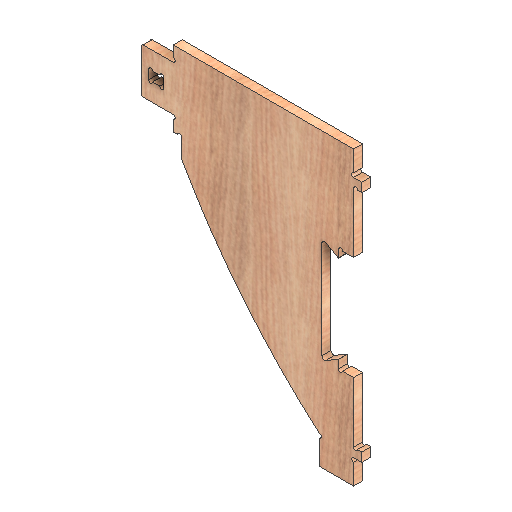
# Autodesk Inventor part: Support F
Saved by Autodesk Inventor 2021 (Build 250183000, 183)
## iProperties
Created: 2020-05-09
Part Number: Support F
Material: Wood (Birch)
Document SubType Name: Modeling
Designer: Dan Wikman
Density: 0.55 g/cm^3
Appearance: Birch - Natural Polished
Mass: 1365.58 g
Surface Area: 3158.08 cm^2
Volume: 2482.87 cm^3
Autodesk Inventor part; units mm, degrees
ref_plane "YZ Plane" through (0, 0, 0) normal (1, 0, 0) x (0, 1, 0)
ref_plane "XZ Plane" through (0, 0, 0) normal (0, 1, 0) x (-1, 0, 0)
ref_plane "XY Plane" through (0, 0, 0) normal (0, 0, 1) x (1, 0, 0)
sketch "CONTOURS" plane through (0, 0, 0) normal (0, 0, 1) x (1, 0, 0)
  arc A0 (2413.107, 689.155) -> (2421.107, 689.155) centre (2417.107, 689.155) ccw
  line L0 (2421.107, 689.155) -> (2429.607, 689.155)
  line L1 (2429.607, 689.155) -> (2429.607, 671.155)
  line L2 (2429.607, 671.155) -> (2413.107, 671.155)
  arc A1 (2413.107, 671.155) -> (2413.107, 663.155) centre (2413.107, 667.155) ccw
  line L3 (2413.107, 663.155) -> (2413.107, 622.1071)
  line L4 (2413.107, 622.1071) -> (2345.607, 622.1071)
  line L5 (2345.607, 622.1071) -> (2345.607, 670.507)
  arc A2 (2345.607, 670.507) -> (2345.607, 678.507) centre (2345.607, 674.507) ccw
  arc A3 (2070.607, 1014.7918) -> (2345.607, 678.507) centre (3181.8457, 1642.9335) ccw
  line L6 (2070.607, 1014.7918) -> (2070.607, 1053.1873)
  arc A4 (2070.607, 1053.1873) -> (2062.607, 1053.1873) centre (2066.607, 1053.1873) ccw
  line L7 (2062.607, 1053.1873) -> (2055.607, 1053.1873)
  line L8 (2055.607, 1053.1873) -> (2054.248, 1053.1873)
  line L9 (2054.248, 1053.1873) -> (2054.248, 1075.1087)
  arc A5 (2054.248, 1075.1087) -> (2054.248, 1083.1087) centre (2054.248, 1079.1087) ccw
  line L10 (2054.248, 1083.1087) -> (1994.248, 1083.1087)
  arc A6 (1990.248, 1087.1087) -> (1994.248, 1083.1087) centre (1994.248, 1087.1087) ccw
  line L11 (1990.248, 1087.1087) -> (1990.248, 1169.1087)
  arc A7 (1994.248, 1173.1087) -> (1990.248, 1169.1087) centre (1994.248, 1169.1087) ccw
  line L12 (1994.248, 1173.1087) -> (2054.248, 1173.1087)
  arc A8 (2054.248, 1173.1087) -> (2054.248, 1181.1087) centre (2054.248, 1177.1087) ccw
  line L13 (2054.248, 1181.1087) -> (2054.248, 1203.107)
  line L14 (2054.248, 1203.107) -> (2413.107, 1203.107)
  line L15 (2413.107, 1203.107) -> (2413.107, 1162.0591)
  arc A9 (2413.107, 1162.0591) -> (2413.107, 1154.0591) centre (2413.107, 1158.0591) ccw
  line L16 (2413.107, 1154.0591) -> (2429.607, 1154.0591)
  line L17 (2429.607, 1154.0591) -> (2429.607, 1136.0591)
  line L18 (2429.607, 1136.0591) -> (2421.107, 1136.0591)
  arc A10 (2421.107, 1136.0591) -> (2413.107, 1136.0591) centre (2417.107, 1136.0591) ccw
  line L19 (2413.107, 1136.0591) -> (2413.107, 1016.107)
  line L20 (2413.107, 1016.107) -> (2391.107, 1016.107)
  arc A11 (2391.107, 1016.107) -> (2383.107, 1016.107) centre (2387.107, 1016.107) ccw
  line L21 (2383.107, 1016.107) -> (2383.107, 999.7176)
  line L22 (2383.107, 999.7176) -> (2382.8653, 999.8478)
  line L23 (2382.8653, 999.8478) -> (2382.6262, 999.9827)
  line L24 (2382.6262, 999.9827) -> (2357.4659, 1014.509)
  arc A12 (2357.4659, 1014.509) -> (2349.9659, 1010.1788) centre (2354.9659, 1010.1788) ccw
  line L25 (2349.9659, 1010.1788) -> (2349.9659, 815.0352)
  arc A13 (2349.9659, 815.0352) -> (2357.4659, 810.7051) centre (2354.9659, 815.0352) ccw
  line L26 (2357.4659, 810.7051) -> (2382.6262, 825.2314)
  line L27 (2382.6262, 825.2314) -> (2382.8653, 825.3663)
  line L28 (2382.8653, 825.3663) -> (2383.107, 825.4965)
  line L29 (2383.107, 825.4965) -> (2383.107, 809.1071)
  arc A14 (2383.107, 809.1071) -> (2391.107, 809.107) centre (2387.107, 809.107) ccw
  line L30 (2391.107, 809.107) -> (2413.107, 809.107)
  line L31 (2413.107, 809.107) -> (2413.107, 689.155)
  constraints: 64 end point, 30 point on circle, 15 centre point
sketch "HOLES" plane through (0, 0, 0) normal (0, 0, 1) x (1, 0, 0)
  arc A0 (2013.248, 1137.6087) -> (2005.248, 1137.6087) centre (2009.248, 1137.6087) ccw
  line L0 (2013.248, 1137.6087) -> (2027.248, 1137.6087)
  arc A1 (2035.248, 1137.6087) -> (2027.248, 1137.6087) centre (2031.248, 1137.6087) ccw
  line L1 (2035.248, 1137.6087) -> (2035.248, 1129.6087)
  line L2 (2035.248, 1129.6087) -> (2035.248, 1118.6087)
  arc A2 (2027.248, 1118.6087) -> (2035.248, 1118.6087) centre (2031.248, 1118.6087) ccw
  line L3 (2027.248, 1118.6087) -> (2013.248, 1118.6087)
  arc A3 (2005.248, 1118.6087) -> (2013.248, 1118.6087) centre (2009.248, 1118.6087) ccw
  line L4 (2005.248, 1118.6087) -> (2005.248, 1129.6087)
  line L5 (2005.248, 1129.6087) -> (2005.248, 1137.6087)
  constraints: 12 end point, 8 point on circle, 4 centre point
sketch "LETTERS" plane through (0, 0, 0) normal (0, 0, 1) x (1, 0, 0)
  line L0 (2183.3626, 1024.3858) -> (2183.3626, 1009.6983)
  line L1 (2183.3626, 1009.6983) -> (2203.1704, 1009.6983)
  line L2 (2193.0627, 1009.6687) -> (2193.0627, 1020.336)
  constraints: 6 end point
extrude "Extrusion3" add sketch "CONTOURS" along normal blind 18
extrude "Extrusion4" cut sketch "HOLES" along normal blind 18
body "Solid2"
